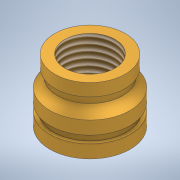
# Autodesk Inventor part: investment nut M2 OD3,2 L2,5
Saved by Autodesk Inventor 2022 (Build 260153000, 153)
## iProperties
Created: 2023-07-18
Part Number: investment nut M2 OD3,2 L2,5
Material: Типовые
Document SubType Name: Modeling
Designer: akapu
Density: 1 g/cm^3
Appearance: По умолчанию
Author: akapu
Autodesk Inventor part; units mm, degrees
ref_plane "YZ Plane" through (0, 0, 0) normal (1, 0, 0) x (0, 1, 0)
ref_plane "XZ Plane" through (0, 0, 0) normal (0, 1, 0) x (-1, 0, 0)
ref_plane "XY Plane" through (0, 0, 0) normal (0, 0, 1) x (1, 0, 0)
sketch "Эскиз1" plane through (0, 0, 0) normal (0, 1, 0) x (-1, 0, 0)
  circle A0 centre (0, 0) radius 1.6
  circle A1 centre (0, 0) radius 1
  dimension "d0" = 3.2
  dimension "d1" = 2
  constraints: 2 centre point, 2 coincident
  measures "d0" diameter of A0
  measures "d1" diameter of A1
extrude "Выдавливание1" add sketch "Эскиз1" along normal blind 2.5
thread "Резьба1" size "M2x0.25" class "6H" standard "ANSI Metric M Profile" length 19.85
sketch "Эскиз2" plane through (0, 0, 0) normal (0, 0, 1) x (1, 0, 0)
  line L0 (1.6, 2.5) -> (-1.6, 2.5) projected
  line L1 (1.6, 2.5) -> (1.3, 2.5)
  line L2 (1.3, 2.5) -> (1.3, 0)
  line L3 (1.6, 0) -> (-1.6, 0) projected
  line L4 (1.6, 2.5) -> (1.6, 0)
  line L5 (0, 0) -> (0, 2.5)
  line L6 (1.6, 2.5) -> (1.6, 2)
  line L7 (1.6, 0) -> (1.6, 2.5) projected
  line L8 (1.6, 2) -> (1.5, 2)
  line L9 (1.5, 2) -> (1.3, 2)
  line L10 (1.3, 2) -> (1.3, 1.7)
  line L11 (1.3, 1.7) -> (1.6, 1.3425)
  line L12 (1.6, 1.3425) -> (1.6, 0)
  line L13 (1.6, 0.6712) -> (1.6, 0.5212)
  line L14 (1.6, 0.5212) -> (1.3, 0.5212)
  line L15 (1.6, 0.6712) -> (1.6, 0.8212)
  line L16 (1.6, 0.8212) -> (1.3, 0.8212)
  line L17 (0, 2.5) -> (1.405, 2.5)
  line L18 (1.405, 2.5) -> (1.4, 2)
  line L19 (0, 0.5212) -> (1.46, 0.5212)
  line L20 (1.46, 0.5212) -> (1.45, 0.8212)
  point P0 (1.6, 0.5212)
  point P1 (1.6, 1.3425)
  dimension "d7" = 0.3
  dimension "d8" = 0.5
  dimension "d10" = 0.3
  dimension "d11" = 40
  dimension "d12" = 0.15
  dimension "d13" = 0.15
  dimension "d15" = 1.405
  dimension "d16" = 1.46
  constraints: 36 end point, 14 point on line, 4 midpoint, 4 perpendicular, 1 collinear, 1 vertical
  measures "d7" distance of L0.start L1.end
  measures "d8" distance of L0.start L6.end
  measures "d10" distance of L9.end L10.end
  measures "d11" angle of L2 L11
  measures "d12" distance of L13.start L13.end
  measures "d13" distance of L13.start L15.end
  measures "d15" distance of L5.end L17.end
  measures "d16" distance of L19.start L19.end
revolve "Вращение1" cut sketch "Эскиз2" angle 360 about axis through (0, 0, 0) along (0, 1, 0) contours L4 L8 L9 L18 L0 | L4 L11 L2 L9 L8 | L4 L14 L20 L16
